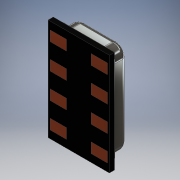
# Autodesk Inventor part: LGA
Saved by Autodesk Inventor 2016 (Build 200138000, 138)
## iProperties
Created: 2016-07-18
Part Number: LGA
Material: Generic
Document SubType Name: Modeling
Designer: Jonathan
Density: 1 g/cm^3
Appearance: Default
Author: Jonathan
Autodesk Inventor part; units mm, degrees
ref_plane "YZ Plane" through (0, 0, 0) normal (1, 0, 0) x (0, 1, 0)
ref_plane "XZ Plane" through (0, 0, 0) normal (0, 1, 0) x (-1, 0, 0)
ref_plane "XY Plane" through (0, 0, 0) normal (0, 0, 1) x (1, 0, 0)
sketch "Sketch1" plane through (0, 0, 0) normal (0, 1, 0) x (-1, 0, 0)
  line L0 (1.5, 2.5) -> (-1.5, 2.5)
  line L1 (-1.5, 2.5) -> (-1.5, -2.5)
  line L2 (-1.5, -2.5) -> (1.5, -2.5)
  line L3 (1.5, -2.5) -> (1.5, 2.5)
  line L4 (1.5, 2.5) -> (-1.5, -2.5) construction
  line L5 (-1.5, 2.5) -> (1.5, -2.5) construction
  point P0 (0, 0)
  dimension "d1" = 3
  dimension "d2" = 5
  constraints: 12 end point, 2 midpoint, 2 parallel, 1 horizontal, 1 perpendicular
  measures "d1" distance of L1.end L2.end
  measures "d2" distance of L0.end L1.end
extrude "Extrusion1" add sketch "Sketch1" along normal blind 0.25
sketch "Sketch2" plane through (0, 0.25, 0) normal (0, 1, 0) x (1, 0, 0)
  line L0 (1.4, -2.4) -> (-1.4, -2.4)
  line L1 (-1.4, -2.4) -> (-1.4, 2.4)
  line L2 (-1.4, 2.4) -> (1.4, 2.4)
  line L3 (1.4, 2.4) -> (1.4, -2.4)
  line L4 (1.4, -2.4) -> (-1.4, 2.4) construction
  line L5 (-1.4, -2.4) -> (1.4, 2.4) construction
  point P0 (0, 0)
  dimension "d5" = 4.8
  dimension "d6" = 2.8
  constraints: 12 end point, 2 midpoint, 2 parallel, 1 horizontal, 1 perpendicular
  measures "d5" distance of L0.end L1.end
  measures "d6" distance of L0.start L0.end
extrude "Extrusion2" add sketch "Sketch2" along normal blind 0.15 separate body
sketch "Sketch3" plane through (0, 0.4, 0) normal (0, 1, 0) x (1, 0, 0)
  line L0 (1.275, -2.275) -> (-1.275, -2.275)
  line L1 (-1.275, -2.275) -> (-1.275, 2.275)
  line L2 (-1.275, 2.275) -> (1.275, 2.275)
  line L3 (1.275, 2.275) -> (1.275, -2.275)
  line L4 (1.275, -2.275) -> (-1.275, 2.275) construction
  line L5 (-1.275, -2.275) -> (1.275, 2.275) construction
  point P0 (0, 0)
  dimension "d9" = 4.55
  dimension "d10" = 2.55
  constraints: 12 end point, 2 midpoint, 2 parallel, 1 horizontal, 1 perpendicular
  measures "d9" distance of L0.end L1.end
  measures "d10" distance of L1.end L2.end
extrude "Extrusion3" add sketch "Sketch3" along normal blind 0.7 bodies 2
sketch "Sketch4" plane through (0, 0, 0) normal (0, -1, 0) x (1, 0, 0)
  line L0 (1.4, -2.125) -> (0.6, -2.125)
  line L1 (0.6, -2.125) -> (0.6, -1.625)
  line L2 (0.6, -1.625) -> (1.4, -1.625)
  line L3 (1.4, -1.625) -> (1.4, -2.125)
  line L4 (1.4, -2.125) -> (0.6, -1.625) construction
  line L5 (0.6, -2.125) -> (1.4, -1.625) construction
  point P0 (0, 0)
  point P1 (1, -1.875)
  dimension "d13" = 0.8
  dimension "d14" = 0.5
  dimension "d15" = 1.875
  dimension "d16" = 1
  constraints: 12 end point, 2 midpoint, 2 parallel, 1 horizontal, 1 perpendicular
  measures "d13" distance of L0.start L0.end
  measures "d14" distance of L2.end L0.start
  measures "d15" vertical distance of point (0, 0) point (1, -1.875)
  measures "d16" horizontal distance of point (0, 0) point (1, -1.875)
extrude "Extrusion4" cut sketch "Sketch4" against normal blind 0.01 bodies 1
pattern_linear "Rectangular Pattern1" count 4 spacing 1.25 along (0, 0, 1) count 2 spacing 2 along (-1, 0, 0) of "Extrusion4" bodies 1
extrude "Extrusion5" add sketch "Sketch4" against normal blind 0.01 separate body
pattern_linear "Rectangular Pattern2" count 4 spacing 1.25 along (0, 0, 1) count 2 spacing 2 along (-1, 0, 0) of "Extrusion5" bodies 3
fillet "Fillet1" radius 0.5 4 edges at (-1.275, 0.75, -2.275) (1.275, 0.75, -2.275) (-1.275, 0.75, 2.275) (1.275, 0.75, 2.275)
fillet "Fillet2" radius 0.3 4 edges at (-1.4, 0.325, -2.4) (1.4, 0.325, -2.4) (-1.4, 0.325, 2.4) (1.4, 0.325, 2.4)
fillet "Fillet4" radius 0.25 8 edges at (-1.1286, 1.1, 2.1286) (0, 1.1, 2.275) (1.1286, 1.1, 2.1286) (1.275, 1.1, 0) (1.1286, 1.1, -2.1286) (0, 1.1, -2.275) (-1.1286, 1.1, -2.1286) (-1.275, 1.1, 0)
fillet "Fillet5" radius 0.05 16 edges at (1.3121, 0.4, 2.3121) (1.4, 0.4, 0) (1.3121, 0.4, -2.3121) (0, 0.4, -2.4) (-1.3121, 0.4, -2.3121) (-1.4, 0.4, 0) (-1.3121, 0.4, 2.3121) (0, 0.4, 2.4) (0, 0.4, 2.275) (1.1286, 0.4, 2.1286) (1.275, 0.4, 0) (1.1286, 0.4, -2.1286) (0, 0.4, -2.275) (-1.1286, 0.4, -2.1286) (-1.275, 0.4, 0) (-1.1286, 0.4, 2.1286)
body "Solid1"
body "Solid2"
body "Solid3"
